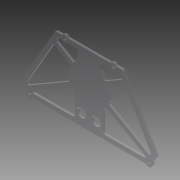
# Autodesk Inventor part: Top Plat
Saved by Autodesk Inventor 2015 (Build 190159000, 159)
## iProperties
Created: 2016-10-14
Part Number: Top Plat
Material: Generic
Document SubType Name: Modeling
Designer: James Yelland
Density: 1 g/cm^3
Appearance: Default
Author: James Yelland
Autodesk Inventor part; units mm, degrees
ref_plane "YZ Plane" through (0, 0, 0) normal (1, 0, 0) x (0, 1, 0)
ref_plane "XZ Plane" through (0, 0, 0) normal (0, 1, 0) x (-1, 0, 0)
ref_plane "XY Plane" through (0, 0, 0) normal (0, 0, 1) x (1, 0, 0)
sketch "Sketch1" plane through (0, 0, 0) normal (0, 1, 0) x (-1, 0, 0)
  circle A0 centre (32.6132, 75.9327) radius 1.6
  circle A1 centre (-32.6132, 75.9327) radius 1.6
  circle A2 centre (80.7596, -11.9856) radius 1.6
  circle A3 centre (-80.7596, -11.9856) radius 1.6
  circle A4 centre (80.7596, -11.9856) radius 5
  circle A5 centre (32.6132, 75.9327) radius 5
  circle A6 centre (-32.6132, 75.9327) radius 5
  circle A7 centre (-80.7596, -11.9856) radius 5
  line L0 (-90.2776, 1.5) -> (-46.4378, 77.4327)
  line L1 (46.4378, 77.4327) -> (90.2776, 1.5)
  line L2 (-83.3494, 1.5) -> (-49.0652, 60.882)
  line L3 (36.6132, 72.9327) -> (40.3756, 72.9327)
  line L4 (48.8642, 61.23) -> (83.3494, 1.5)
  line L5 (83.3494, -1.5) -> (83.1439, -1.8558)
  line L6 (85.3577, -10.0215) -> (90.2776, -1.5)
  line L7 (43.8397, 78.9327) -> (36.6132, 78.9327)
  line L8 (-28.6132, 78.9327) -> (28.6132, 78.9327)
  line L9 (-36.6132, 72.9327) -> (-40.3756, 72.9327)
  line L10 (-36.6132, 78.9327) -> (-43.8397, 78.9327)
  line L11 (-83.3494, -1.5) -> (-83.1439, -1.8558)
  line L12 (-85.3577, -10.0215) -> (-90.2776, -1.5)
  line L13 (-80.7596, -11.9856) -> (-77.7596, -11.9856) construction
  line L14 (76.7596, -14.9856) -> (-76.7596, -14.9856)
  arc A8 (90.2776, -1.5) -> (90.2776, 1.5) centre (87.6795, 0) ccw
  arc A9 (83.3494, -1.5) -> (83.3494, 1.5) centre (80.7513, 0) ccw
  arc A10 (46.4378, 77.4327) -> (43.8397, 78.9327) centre (43.8397, 75.9327) ccw
  arc A11 (42.9737, 71.4327) -> (40.3756, 72.9327) centre (40.3756, 69.9327) ccw
  arc A12 (-43.8397, 78.9327) -> (-46.4378, 77.4327) centre (-43.8397, 75.9327) ccw
  arc A13 (-40.3756, 72.9327) -> (-42.9737, 71.4327) centre (-40.3756, 69.9327) ccw
  arc A14 (-83.3494, 1.5) -> (-83.3494, -1.5) centre (-80.7513, 0) ccw
  arc A15 (-90.2776, 1.5) -> (-90.2776, -1.5) centre (-87.6795, 0) ccw
  line L15 (42.9737, 71.4327) -> (44.3642, 69.0243)
  line L16 (-42.9737, 71.4327) -> (-44.5652, 68.6762)
  line L17 (8.4338, -14.9856) -> (23.4338, -14.9856)
  line L18 (66.4338, -8.9856) -> (74.8949, -8.9856)
  circle A16 centre (-10, 1.1144) radius 6.25
  circle A17 centre (10, 1.1144) radius 6.25
  line L19 (66.4338, -8.9856) -> (22, -8.9856)
  line L20 (-74.8949, -8.9856) -> (-22, -8.9856)
  line L21 (-19, -5.9856) -> (-19, 16.3195)
  line L22 (19, -5.9856) -> (19, 16.3195)
  arc A18 (-22, -8.9856) -> (-19, -5.9856) centre (-22, -5.9856) ccw
  arc A19 (19, -5.9856) -> (22, -8.9856) centre (22, -5.9856) ccw
  line L23 (15.2998, 64.5183) -> (15.2998, 69.9327)
  line L24 (-15.2998, 64.5183) -> (-15.2998, 69.9327)
  line L25 (28.6132, 72.9327) -> (18.2998, 72.9327)
  line L26 (-18.2998, 72.9327) -> (-28.6132, 72.9327)
  arc A20 (29.7335, 35.7144) -> (29.7335, 38.7144) centre (27.1355, 37.2144) ccw
  arc A21 (19.4019, 17.8195) -> (19, 16.3195) centre (22, 16.3195) ccw
  arc A22 (-19, 16.3195) -> (-19.4019, 17.8195) centre (-22, 16.3195) ccw
  arc A23 (-29.7335, 38.7144) -> (-29.7335, 35.7144) centre (-27.1355, 37.2144) ccw
  arc A24 (-15.7017, 63.0183) -> (-15.2998, 64.5183) centre (-18.2998, 64.5183) ccw
  arc A25 (-15.2998, 69.9327) -> (-18.2998, 72.9327) centre (-18.2998, 69.9327) ccw
  arc A26 (18.2998, 72.9327) -> (15.2998, 69.9327) centre (18.2998, 69.9327) ccw
  line L27 (25.3157, 49.3664) -> (46.8152, 61.7791)
  line L28 (22.3157, 54.5625) -> (43.8152, 66.9752)
  line L29 (-25.5167, 49.0183) -> (-47.0161, 61.431)
  line L30 (-22.5167, 54.2144) -> (-44.0161, 66.6272)
  line L31 (27.3668, 28.6151) -> (81.0949, -2.4049)
  line L32 (24.3668, 23.4189) -> (75.6449, -6.1865)
  line L33 (-24.3668, 23.4189) -> (-75.6449, -6.1865)
  line L34 (-27.3668, 28.6151) -> (-81.0949, -2.4049)
  line L35 (-15.7017, 63.0183) -> (-20.4676, 54.7635)
  line L36 (-24.9676, 46.9692) -> (-29.7335, 38.7144)
  line L37 (-29.7335, 35.7144) -> (-26.8177, 30.6641)
  line L38 (-22.3177, 22.8699) -> (-19.4019, 17.8195)
  arc A27 (15.2998, 64.5183) -> (15.7017, 63.0183) centre (18.2998, 64.5183) ccw
  line L39 (15.7017, 63.0183) -> (20.2667, 55.1115)
  line L40 (24.7667, 47.3173) -> (29.7335, 38.7144)
  line L41 (29.7335, 35.7144) -> (26.8177, 30.6641)
  line L42 (22.3177, 22.8699) -> (19.4019, 17.8195)
  arc A28 (20.2667, 55.1115) -> (22.3157, 54.5625) centre (21.5657, 55.8615) ccw
  arc A29 (25.3157, 49.3664) -> (24.7667, 47.3173) centre (26.0657, 48.0673) ccw
  arc A30 (26.8177, 30.6641) -> (27.3668, 28.6151) centre (28.1168, 29.9141) ccw
  arc A31 (24.3668, 23.4189) -> (22.3177, 22.8699) centre (23.6168, 22.1199) ccw
  arc A32 (-24.9676, 46.9692) -> (-25.5167, 49.0183) centre (-26.2667, 47.7192) ccw
  arc A33 (-22.5167, 54.2144) -> (-20.4676, 54.7635) centre (-21.7667, 55.5135) ccw
  arc A34 (-27.3668, 28.6151) -> (-26.8177, 30.6641) centre (-28.1168, 29.9141) ccw
  arc A35 (-22.3177, 22.8699) -> (-24.3668, 23.4189) centre (-23.6168, 22.1199) ccw
  arc A36 (81.0949, -2.4049) -> (83.1439, -1.8558) centre (81.8449, -1.1058) ccw
  arc A37 (48.8642, 61.23) -> (46.8152, 61.7791) centre (47.5652, 60.48) ccw
  arc A38 (43.8152, 66.9752) -> (44.3642, 69.0243) centre (43.0652, 68.2743) ccw
  arc A39 (-83.1439, -1.8558) -> (-81.0949, -2.4049) centre (-81.8449, -1.1058) ccw
  arc A40 (-47.0161, 61.431) -> (-49.0652, 60.882) centre (-47.7661, 60.132) ccw
  arc A41 (-44.5652, 68.6762) -> (-44.0161, 66.6272) centre (-43.2661, 67.9262) ccw
  arc A42 (74.8949, -8.9856) -> (75.6449, -6.1865) centre (74.8949, -7.4856) ccw
  arc A43 (-75.6449, -6.1865) -> (-74.8949, -8.9856) centre (-74.8949, -7.4856) ccw
  point P0 (45.5718, 78.9327)
  point P1 (91.1436, 0)
  point P2 (-84.2154, 0)
  point P3 (-42.1077, 72.9327)
  point P4 (80.1615, -7.0215)
  point P5 (-80.1615, -7.0215)
  point P6 (76.7596, -8.9856)
  point P7 (45.4737, 67.1025)
  point P8 (-80.8494, -5.8301)
  point P9 (48.4737, 61.9064)
  point P10 (-74.3148, -8.9856)
  point P11 (-45.3152, 67.3772)
  point P12 (80.8494, -5.8301)
  point P13 (-48.4737, 61.9064)
  point P14 (74.3148, -8.9856)
  point P15 (-66.2073, 31.191)
  point P16 (-76.7596, -8.9856)
  point P17 (-19, -8.9856)
  point P18 (19, 14.2144)
  point P19 (-19, 14.2144)
  point P20 (0, 37.2144)
  point P21 (30.5996, 37.2144)
  point P22 (-30.5996, 37.2144)
  point P23 (-15.2998, 63.7144)
  point P24 (15.2998, 63.7144)
  point P25 (48.1142, 62.5291)
  point P26 (-48.3152, 62.181)
  point P27 (78.2245, -7.6759)
  point P28 (-78.2245, -7.6759)
  dimension "d2" = 3.2
  dimension "d24" = 3
  dimension "d93" = 3
  dimension "d94" = 1.5
  dimension "d95" = 1.5
  constraints: 86 end point, 86 point on circle, 60 tangent, 44 centre point, 36 point on line, 27 equal radius, 4 coincident, 4 collinear, 3 horizontal, 3 perpendicular, 2 parallel, 2 vertical, 1 midpoint, 4 other
  measures "d2" diameter of A3
  measures "d24" radius of A8
  measures "d93" radius of A27
  measures "d94" radius of A28
  measures "d95" radius of A42
extrude "Extrusion1" add sketch "Sketch1" along normal blind 3 contours A4 | A4 L14 A7 L12 A15 L0 A12 L10 A6 L9 A13 L16 A41 L30 A33 L35 A24 L24 A25 L26 L8 A5 L25 A26 L23 A27 L39 A28 L28 A38 L15 A11 L3 L7 A10 L1 A8 L6 | A7 | A5 | A6
body "Solid1"
